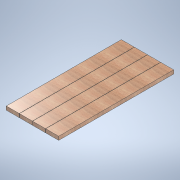
# Autodesk Inventor part: Desk Top Secondary
Saved by Autodesk Inventor 2020.2 (Build 242310000, 310)
## iProperties
Created: 2019-12-30
Part Number: Desk Top Secondary
Material: Wood (Birch - Stained)
Document SubType Name: Modeling
Designer: Andrew
Density: 0.1 g/cm^3
Appearance: Birch - Stained Light
l_2x4: 96.000 in
w_2x4: 3.585 in
h_2x4: 1.563 in
l_2x6: 96.000 in
w_2x6: 5.643 in
h_2x6: 1.563 in
plank_tol: 0.063 in
Author: Andrew
Autodesk Inventor part; units mm, degrees
ref_plane "YZ Plane" through (0, 0, 0) normal (1, 0, 0) x (0, 1, 0)
ref_plane "XZ Plane" through (0, 0, 0) normal (0, 1, 0) x (-1, 0, 0)
ref_plane "XY Plane" through (0, 0, 0) normal (0, 0, 1) x (1, 0, 0)
derived "Desk Top Primary.ipt"
sketch "Ideal" plane through (0, 0, 0) normal (0, 1, 0) x (-1, 0, 0)
  line L0 (0, 0) -> (-2438.4, 0)
  line L1 (-2438.4, 0) -> (-2438.4, 609.6)
  line L2 (-2438.4, 609.6) -> (-609.6, 609.6)
  line L3 (-609.6, 609.6) -> (-609.6, 1219.2)
  line L4 (-609.6, 1219.2) -> (0, 1219.2)
  line L5 (0, 1219.2) -> (0, 0)
sketch "Primary Top" plane through (0, 0, 0) normal (0, 1, 0) x (-1, 0, 0)
  line L0 (-2713.228, 0) -> (-579.628, 0)
  line L1 (-579.628, 0) -> (-579.628, 143.3195)
  line L2 (-579.628, 143.3195) -> (-2713.228, 143.3195)
  line L3 (-2713.228, 143.3195) -> (-2713.228, 0)
  line L4 (-2713.228, 144.907) -> (-579.628, 144.907)
  line L5 (-579.628, 144.907) -> (-579.628, 288.2265)
  line L6 (-579.628, 288.2265) -> (-2713.228, 288.2265)
  line L7 (-2713.228, 288.2265) -> (-2713.228, 144.907)
  line L8 (-2713.228, 289.814) -> (-579.628, 289.814)
  line L9 (-579.628, 289.814) -> (-579.628, 433.1335)
  line L10 (-579.628, 433.1335) -> (-2713.228, 433.1335)
  line L11 (-2713.228, 433.1335) -> (-2713.228, 289.814)
  line L12 (-2713.228, 434.721) -> (-579.628, 434.721)
  line L13 (-579.628, 434.721) -> (-579.628, 578.0405)
  line L14 (-579.628, 578.0405) -> (-2713.228, 578.0405)
  line L15 (-2713.228, 578.0405) -> (-2713.228, 434.721)
  point P0 (0, 0)
sketch "Secondary Top" plane through (0, 0, 0) normal (0, 1, 0) x (-1, 0, 0)
  line L0 (0, 1270) -> (-143.3195, 1270)
  line L1 (-143.3195, 1270) -> (-143.3195, 0)
  line L2 (-143.3195, 0) -> (0, 0)
  line L3 (0, 0) -> (0, 1270)
  line L4 (-144.907, 1270) -> (-288.2265, 1270)
  line L5 (-288.2265, 1270) -> (-288.2265, 0)
  line L6 (-288.2265, 0) -> (-144.907, 0)
  line L7 (-144.907, 0) -> (-144.907, 1270)
  line L8 (-289.814, 1270) -> (-433.1335, 1270)
  line L9 (-433.1335, 1270) -> (-433.1335, 0)
  line L10 (-433.1335, 0) -> (-289.814, 0)
  line L11 (-289.814, 0) -> (-289.814, 1270)
  line L12 (-434.721, 1270) -> (-578.0405, 1270)
  line L13 (-578.0405, 1270) -> (-578.0405, 0)
  line L14 (-578.0405, 0) -> (-434.721, 0)
  line L15 (-434.721, 0) -> (-434.721, 1270)
  dimension "d1" = 143.3195
  dimension "d2" = 143.3195
  dimension "d3" = 143.3195
  dimension "d4" = 143.3195
  dimension "d5" = 1.5875
  dimension "d6" = 1.5875
  dimension "d7" = 1.5875
  dimension "d8" = 1270
  constraints: 32 end point, 8 parallel, 6 point on line, 4 horizontal, 4 perpendicular, 1 coincident
  measures "d1" distance of L0.start L0.end
  measures "d2" distance of L4.start L4.end
  measures "d3" distance of L8.start L8.end
  measures "d4" distance of L12.start L12.end
  measures "d5" distance between parallel lines of L7 L1
  measures "d6" distance between parallel lines of L11 L5
  measures "d7" distance between parallel lines of L15 L9
  measures "d8" distance of L2.end L0.start
extrude "Extrusion1" add sketch "Secondary Top" along normal blind 39.6966
equation "\"d1\" = w_2x6"
equation "\"d2\" = d1"
equation "\"d3\" = d1"
equation "\"d4\" = d1"
equation "\"d5\" = plank_tol"
equation "\"d6\" = plank_tol"
equation "\"d7\" = plank_tol"
equation "\"d9\" = h_2x6"
equation "\"w_2x6\" = 143.3195"
equation "\"plank_tol\" = 1.5875"
equation "\"h_2x6\" = 39.696571"
body "Solid1"
